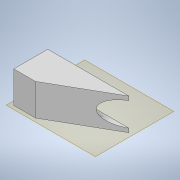
# Autodesk Inventor part: Wire_Clossing
Saved by Autodesk Inventor 2022.3 (Build 263350000, 350)
## iProperties
Created: 2023-05-07
Part Number: Wire_Clossing
Material: Generic
Document SubType Name: Modeling
Designer: Manuel Hueso Béjar
Density: 1 g/cm^3
Appearance: Default
Author: Manuel Hueso Béjar
Autodesk Inventor part; units mm, degrees
ref_plane "YZ Plane" through (0, 0, 0) normal (1, 0, 0) x (0, 1, 0)
ref_plane "XZ Plane" through (0, 0, 0) normal (0, 1, 0) x (-1, 0, 0)
ref_plane "XY Plane" through (0, 0, 0) normal (0, 0, 1) x (1, 0, 0)
ref_plane "Work Plane1" through (-6.4883, -6.1632, -131.5017) normal (0, 1, 0) x (-1, 0, 0)
sketch "Sketch1" plane through (-6.4883, -6.1632, -131.5017) normal (0, 1, 0) x (-1, 0, 0)
  line L0 (-2, -18) -> (-2, 0) projected
  line L1 (-2, 0) -> (-7.4816, 0) projected
  line L2 (-22.4693, -8.5807) -> (-7.4816, 0) projected
  line L3 (-6.2906, -18) -> (-22.4693, -8.5807) projected
  line L4 (-2, -18) -> (-6.2906, -18) projected
  point P0 (-6.4883, 131.5017)
extrude "Extrusion1" add sketch "Sketch1" along normal blind 8
sketch "Sketch2" plane through (0, 0, 0) normal (1, 0, 0) x (0, 1, 0)
  line L0 (-6.1632, -140.0824) -> (1.8368, -140.0824) projected
  circle A0 centre (-2.1632, -140.0824) radius 3
  point P0 (0, 0)
  dimension "d2" = 6
  constraints: 1 centre point, 1 midpoint
  measures "d2" diameter of A0
extrude "Extrusion2" cut sketch "Sketch2" along normal through all both and the other way through all
sketch "Sketch3" plane through (-6.4883, 1.8368, -131.5017) normal (0, 1, 0) x (1, 0, 0)
  line L0 (6.2906, 18) -> (2, 18) projected
  line L1 (17.3164, 11.5807) -> (22.4693, 8.5807) projected
  line L2 (2, 18) -> (22.4693, 18)
  line L3 (22.4693, 18) -> (22.4693, 8.5807)
  line L4 (22.4693, 8.5807) -> (2, 8.5807)
  line L5 (2, 8.5807) -> (2, 18)
  point P0 (6.4883, -131.5017)
  constraints: 8 end point, 2 parallel, 1 horizontal, 1 perpendicular
extrude "Extrusion3" cut sketch "Sketch3" against normal through all
body "Solid1"
